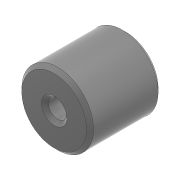
# Autodesk Inventor part: spacerwiel
Saved by Autodesk Inventor 2020.3 (Build 243373000, 373)
## iProperties
Created: 2020-10-19
Part Number: spacerwiel
Material: ABS Plastic
Document SubType Name: Modeling
Designer: Svend
Density: 1.06 g/cm^3
Appearance: Smooth - White
Author: Svend
Autodesk Inventor part; units mm, degrees
ref_plane "YZ Plane" through (0, 0, 0) normal (1, 0, 0) x (0, 1, 0)
ref_plane "XZ Plane" through (0, 0, 0) normal (0, 1, 0) x (-1, 0, 0)
ref_plane "XY Plane" through (0, 0, 0) normal (0, 0, 1) x (1, 0, 0)
sketch "Sketch1" plane through (0, 0, 0) normal (0, 0, 1) x (1, 0, 0)
  circle A0 centre (0, 0) radius 20
  circle A1 centre (0, 0) radius 5.1
  dimension "d0" = 40
  dimension "d1" = 10.2
  constraints: 2 centre point, 2 coincident
  measures "d0" diameter of A0
  measures "d1" diameter of A1
extrude "Extrusion1" add sketch "Sketch1" along normal blind 40
chamfer "Chamfer1" distance 2 angle 45 4 edges at (-20, 0, 0) (-20, 0, 40) (-5.1, 0, 0) (-5.1, 0, 40)
body "Solid1"
